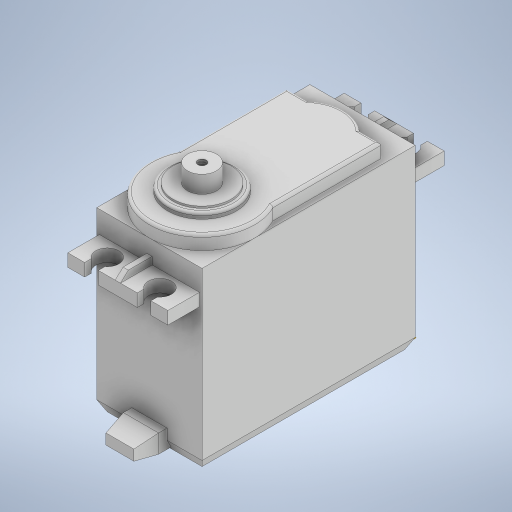
# Autodesk Inventor part: Hitec HS-425BB Servo
Saved by Autodesk Inventor 2023 (Build 270158000, 158)
## iProperties
Created: 2023-09-01
Part Number: Hitec HS-425BB Servo
Material: Generic
Document SubType Name: Modeling
Designer: Nate
Density: 1 g/cm^3
Appearance: Default
Author: Nate
Autodesk Inventor part; units mm, degrees
ref_plane "YZ Plane" through (0, 0, 0) normal (1, 0, 0) x (0, 1, 0)
sketch "Sketch1" plane through (0, 0, 0) normal (0, 1, 0) x (-1, 0, 0)
  line L0 (0, 0) -> (20, 0)
  line L1 (20, 0) -> (20, 40.5)
  line L2 (20, 40.5) -> (0, 40.5)
  line L3 (0, 40.5) -> (0, 0)
  line L4 (6.65, 40.5) -> (13.35, 40.5)
  line L5 (13.35, 40.5) -> (13.35, 42.1)
  line L6 (13.35, 42.1) -> (6.65, 42.1)
  line L7 (6.65, 42.1) -> (6.65, 40.5)
  line L8 (6.65, 42.1) -> (13.35, 42.1)
  line L9 (13.35, 42.1) -> (13.35, 46.1)
  line L10 (13.35, 46.1) -> (6.65, 46.1)
  line L11 (6.65, 46.1) -> (6.65, 42.1)
  point P0 (13.35, 41.3)
  point P1 (6.65, 41.3)
  dimension "d1" = 40.5
  dimension "d2" = 1.6
  dimension "d3" = 6.7
  dimension "d5" = 6.65
  dimension "d6" = 6.7
  dimension "d7" = 4
  dimension "d8" = 20
  constraints: 24 end point, 6 parallel, 3 horizontal, 3 perpendicular, 2 midpoint, 1 point on line
  measures "d1" distance of L1.end L0.end
  measures "d2" distance of L5.end L4.end
  measures "d3" distance of point (13.35, 41.3) point (6.65, 41.3)
  measures "d5" horizontal distance of point (6.65, 41.3) L2.end
  measures "d6" distance of L10.end L9.end
  measures "d7" distance of L9.end L8.end
  measures "d8" distance between parallel lines of L3 L1
extrude "Extrusion1" add sketch "Sketch1" along normal blind 31.6 and the other way blind 2 contours L3 L2 L1 L0
extrude "Extrusion2" add sketch "Sketch1" along normal blind 2 and the other way blind 1.5 contours L7 L6 L5 L2 | L11 L10 L9 L6
chamfer "Chamfer1" distance 4 distance2 1 1 edges at (-10, 2, 46.1) measured on face at (-10, 2, 45.6)
chamfer "Chamfer2" distance 4 distance2 0.5 1 edges at (-10, -1.5, 46.1) measured on face at (-10, -1.5, 45.6)
chamfer "Chamfer3" distance 4 distance2 0.7 1 edges at (-13.35, 0, 46.1) measured on face at (-13.35, 0, 45.6)
chamfer "Chamfer4" distance 0.7 distance2 4 1 edges at (-6.65, 0, 46.1) measured on face at (-7.15, 0, 46.1)
chamfer "Chamfer5" distance 1 angle 63.4 4 edges at (0, -2, 20.25) (-10, -2, 0) (-20, -2, 20.25) (-10, -2, 40.5) measured on face at (-10, -2, 0.5) measured on face at (-10, -2, 40) measured on face at (-19.5, -2, 20.25) measured on face at (-0.5, -2, 20.25)
ref_plane "Work Plane1" through (0, 25.02, 0) normal (0, 1, 0) x (-1, 0, 0)
sketch "Sketch2" plane through (0, 25.02, 0) normal (0, 1, 0) x (-1, 0, 0)
  line L0 (20, 40.5) -> (0, 40.5) projected
  line L1 (0.5, 40.5) -> (19.5, 40.5)
  line L2 (19.5, 40.5) -> (19.5, 46.5)
  line L3 (19.5, 46.5) -> (0.5, 46.5)
  line L4 (0.5, 46.5) -> (0.5, 40.5)
  line L5 (0, 40.5) -> (0, 0) projected
  line L6 (3.7, 46.5) -> (6.3, 46.5)
  line L7 (6.3, 46.5) -> (6.3, 43.5)
  line L8 (6.3, 43.5) -> (3.7, 43.5)
  line L9 (3.7, 43.5) -> (3.7, 46.5)
  line L10 (16.3, 46.5) -> (13.7, 46.5)
  line L11 (13.7, 46.5) -> (13.7, 43.5)
  line L12 (13.7, 43.5) -> (16.3, 43.5)
  line L13 (16.3, 43.5) -> (16.3, 46.5)
  circle A0 centre (15, 43.5) radius 2.18
  circle A1 centre (5, 43.5) radius 2.18
  line L14 (10.5, 46.5) -> (9.5, 46.5)
  line L15 (9.5, 46.5) -> (9.5, 40.5)
  line L16 (9.5, 40.5) -> (10.5, 40.5)
  line L17 (10.5, 40.5) -> (10.5, 46.5)
  line L18 (9.5, 46.5) -> (10.5, 46.5)
  line L19 (10.5, 46.5) -> (9.5, 46.5)
  point P0 (3.7, 45)
  point P1 (16.3, 45)
  point P2 (10, 40.5)
  point P3 (10, 46.5)
  point P4 (10, 46.5)
  point P5 (6.3, 45.25)
  point P6 (3.7, 45.25)
  point P7 (16.3, 45.25)
  point P8 (13.7, 45.25)
  dimension "d33" = 19
  dimension "d34" = 6
  dimension "d35" = 0.5
  dimension "d36" = 2.6
  dimension "d37" = 3
  dimension "d38" = 2.6
  dimension "d39" = 3
  dimension "d40" = 3.2
  dimension "d41" = 3.2
  dimension "d42" = 4.36
  dimension "d43" = 3
  dimension "d44" = 15
  dimension "d45" = 4.36
  dimension "d46" = 3
  dimension "d47" = 5
  dimension "d48" = 1
  dimension "d49" = 6
  dimension "d50" = 9.5
  constraints: 36 end point, 9 equal length, 7 midpoint, 5 horizontal, 4 perpendicular, 4 point on line, 2 centre point
  measures "d33" distance of L3.end L2.end
  measures "d34" distance of L2.end L1.end
  measures "d35" distance between parallel lines of L5 L4
  measures "d36" distance of L7.end L8.end
  measures "d37" distance of L6.end L7.end
  measures "d38" distance of L12.end L11.end
  measures "d39" distance of L11.end L10.end
  measures "d40" distance from line of point (3.7, 45) L4
  measures "d41" distance from line of L2 point (16.3, 45)
  measures "d42" diameter of A0
  measures "d43" distance from line of L0 A0.centre
  measures "d44" distance from line of L5 A0.centre
  measures "d45" diameter of A1
  measures "d46" distance from line of L1 A1.centre
  measures "d47" distance from line of L5 A1.centre
  measures "d48" distance of L16.end L15.end
  measures "d49" distance of L15.end L14.end
  measures "d50" distance between parallel lines of L5 L15
extrude "Extrusion3" add sketch "Sketch2" along normal blind 2.4 contours L0 L17 L3 L11 A0 L13 L2 | L0 L4 L3 L9 A1 L7 L15
extrude "Extrusion4" add sketch "Sketch2" along normal blind 3.8 contours L0 L15 L3 L17
ref_plane "Work Plane2" through (0, 0, 20.25) normal (0, 0, 1) x (1, 0, 0)
mirror "Mirror1" about plane through (0, 0, 20.25) normal (0, 0, 1) of "Extrusion3", "Extrusion4"
chamfer "Chamfer7" distance 1.5 distance2 1.4 1 edges at (-10, 28.82, 46.5) measured on face at (-10, 28.82, 46)
chamfer "Chamfer8" distance 1.5 distance2 1.4 1 edges at (-10, 28.82, -6) measured on face at (-10, 28.82, -5.5)
sketch "Sketch3" plane through (0, 31.6, 0) normal (0, 1, 0) x (1, 0, 0)
  line L0 (-18.93, -30.5) -> (-1.07, -30.5)
  line L1 (-1.07, -30.5) -> (-1.07, -5.5)
  line L2 (-1.07, -5.5) -> (-18.93, -5.5)
  line L3 (-18.93, -5.5) -> (-18.93, -30.5)
  line L4 (0, -40.5) -> (0, 0) projected
  line L5 (-20, -40.5) -> (0, -40.5) projected
  line L6 (-20, -40.5) -> (0, -40.5) projected
  line L7 (0, -40.5) -> (0, 0) projected
  line L8 (0, 0) -> (-20, 0) projected
  line L9 (-20, 0) -> (-20, -40.5) projected
  circle A0 centre (-10, -11.02) radius 7.4
  circle A1 centre (-10, -30.5) radius 6.5
  circle A2 centre (-10, -30.5) radius 2.75
  circle A3 centre (-10, -30.5) radius 5.5
  circle A4 centre (-10, -30.5) radius 10
  point P0 (-10, -40.5)
  point P1 (-1.07, -25.9994)
  point P2 (-5.0716, -5.5)
  point P3 (-14.9284, -5.5)
  point P4 (-18.93, -25.9994)
  dimension "d69" = 1.07
  dimension "d70" = 18.93
  dimension "d71" = 10
  dimension "d72" = 35
  dimension "d73" = 14.8
  dimension "d74" = 29.48
  dimension "d75" = 13
  dimension "d76" = 10
  dimension "d77" = 10
  dimension "d78" = 10
  dimension "d79" = 5.5
  dimension "d80" = 11
  dimension "d81" = 20
  constraints: 8 end point, 5 centre point, 3 coincident, 2 parallel, 1 horizontal, 1 midpoint, 1 perpendicular
  measures "d69" distance between parallel lines of L1 L4
  measures "d70" distance between parallel lines of L4 L3
  measures "d71" distance between parallel lines of L0 L5
  measures "d72" distance between parallel lines of L2 L5
  measures "d73" diameter of A0
  measures "d74" distance from line of A0.centre L5
  measures "d75" diameter of A1
  measures "d76" distance of A1.centre point (-10, -40.5)
  measures "d77" distance from line of A1.centre L4
  measures "d78" distance from line of L4 A0.centre
  measures "d79" diameter of A2
  measures "d80" diameter of A3
  measures "d81" diameter of A4
extrude "Extrusion5" add sketch "Sketch3" along normal blind 2.68 contours A1 L0 L3 A4 L1 | L0 L1 A4 L3 A1 | A4 L3 L2 A0 L1 | A0 L2 | L2 A0
extrude "Extrusion6" add sketch "Sketch3" along normal blind 3.78 contours A2 L0 A3 | A2 L0 | L0 A2 | L0 A3 A2 | A3 L0 A1 | L0 A1 A3
extrude "Extrusion7" add sketch "Sketch3" along normal blind 4.13 contours A2 L0 A3 | L0 A3 A2
extrude "Extrusion8" add sketch "Sketch3" along normal blind 7.43 contours A2 L0 | L0 A2
sketch "Sketch4" plane through (-10, 39.03, 30.5) normal (0, 1, 0) x (1, 0, 0)
  circle A0 centre (0, 0) radius 0.2
  point P0 (10, 30.5)
  dimension "d90" = 0.4
  constraints: 1 centre point
  measures "d90" diameter of A0
hole "Hole1" at (-10, 39.03, 30.5) direction (0, -1, 0) diameter 1.567 depth 6 tip angle 118 thread size "M2x0.4" class "6H" standard "ISO Metric profile"
fillet "Fillet1" radius 0.5 1 edges at (-16.5, 35.38, 30.5)
fillet "Fillet2" radius 0.5 6 edges at (-18.93, 34.28, 15.7497) (-10, 34.28, 40.5) (-1.07, 34.28, 15.7497) (-3.0708, 34.28, 5.5) (-10, 34.28, 3.62) (-16.9292, 34.28, 5.5)
body "Solid1"
